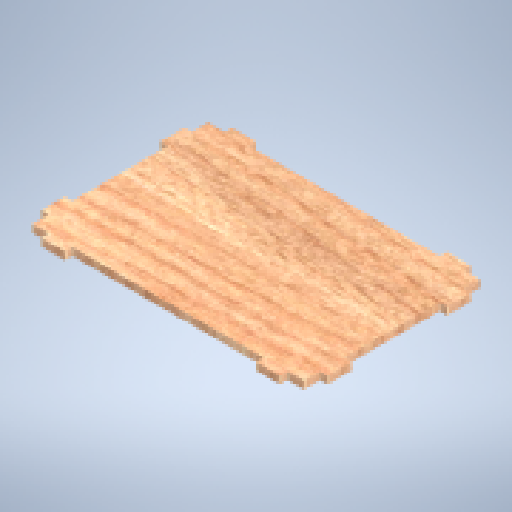
# Autodesk Inventor part: Bottom Panel
Saved by Autodesk Inventor 2023.1 (Build 271208000, 208)
## iProperties
Created: 2022-07-14
Part Number: Bottom Panel
Material: Wood (Birch)
Document SubType Name: Modeling
Designer: Eli
Density: 0.55 g/cm^3
Appearance: Birch - Natural Polished
Author: Eli
Autodesk Inventor part; units mm, degrees
ref_plane "YZ Plane" through (0, 0, 0) normal (1, 0, 0) x (0, 1, 0)
ref_plane "XZ Plane" through (0, 0, 0) normal (0, 1, 0) x (-1, 0, 0)
ref_plane "XY Plane" through (0, 0, 0) normal (0, 0, 1) x (1, 0, 0)
sketch "Sketch1" plane through (0, 0, 0) normal (0, 1, 0) x (-1, 0, 0)
  line L0 (0, 0) -> (152.4, 0)
  line L1 (152.4, 0) -> (152.4, 101.6)
  line L2 (152.4, 101.6) -> (0, 101.6)
  line L3 (0, 101.6) -> (0, 0)
  line L4 (152.4, 0) -> (139.7, 0)
  line L5 (139.7, 0) -> (139.7, 4)
  line L6 (139.7, 4) -> (152.4, 4)
  line L7 (152.4, 4) -> (152.4, 0)
  line L8 (0, 0) -> (12.7, 0)
  line L9 (12.7, 0) -> (12.7, 4)
  line L10 (12.7, 4) -> (0, 4)
  line L11 (0, 4) -> (0, 0)
  line L12 (127, 0) -> (25.4, 0)
  line L13 (25.4, 0) -> (25.4, 4)
  line L14 (25.4, 4) -> (127, 4)
  line L15 (127, 4) -> (127, 0)
  line L16 (152.4, 50.8) -> (0, 50.8)
  line L17 (139.7, 101.6) -> (139.7, 97.6)
  line L18 (139.7, 97.6) -> (152.4, 97.6)
  line L19 (12.7, 101.6) -> (12.7, 97.6)
  line L20 (12.7, 97.6) -> (0, 97.6)
  line L21 (25.4, 101.6) -> (25.4, 97.6)
  line L22 (25.4, 97.6) -> (127, 97.6)
  line L23 (127, 97.6) -> (127, 101.6)
  line L24 (152.4, 101.6) -> (148.4, 101.6)
  line L25 (148.4, 101.6) -> (148.4, 88.9)
  line L26 (148.4, 88.9) -> (152.4, 88.9)
  line L27 (152.4, 88.9) -> (152.4, 101.6)
  line L28 (152.4, 0) -> (148.4, 0)
  line L29 (148.4, 0) -> (148.4, 12.7)
  line L30 (148.4, 12.7) -> (152.4, 12.7)
  line L31 (152.4, 12.7) -> (152.4, 0)
  line L32 (152.4, 76.2) -> (148.4, 76.2)
  line L33 (148.4, 76.2) -> (148.4, 25.4)
  line L34 (148.4, 25.4) -> (152.4, 25.4)
  line L35 (152.4, 25.4) -> (152.4, 76.2)
  line L36 (76.2, 97.6) -> (76.2, 4)
  line L37 (4, 101.6) -> (4, 88.9)
  line L38 (4, 88.9) -> (0, 88.9)
  line L39 (4, 0) -> (4, 12.7)
  line L40 (4, 12.7) -> (0, 12.7)
  line L41 (0, 76.2) -> (4, 76.2)
  line L42 (4, 76.2) -> (4, 25.4)
  line L43 (4, 25.4) -> (0, 25.4)
  point P0 (12.7, 2)
  point P1 (25.4, 2)
  point P2 (150.4, 12.7)
  point P3 (150.4, 25.4)
  point P4 (150.4, 88.9)
  point P5 (150.4, 76.2)
  point P6 (148.4, 97.6)
  point P7 (4, 97.6)
  point P8 (4, 4)
  point P9 (25.4, 0)
  point P10 (148.4, 4)
  dimension "d0" = 152.4
  dimension "d1" = 101.6
  dimension "d2" = 12.7
  dimension "d3" = 4
  dimension "d4" = 12.7
  dimension "d5" = 4
  dimension "d6" = 4
  dimension "d7" = 12.7
  dimension "d8" = 12.7
  dimension "d9" = 4
  dimension "d10" = 12.7
  dimension "d11" = 4
  dimension "d12" = 12.7
  dimension "d13" = 4
  dimension "d14" = 12.7
  dimension "d15" = 12.7
  constraints: 88 end point, 20 symmetric about line, 14 parallel, 10 midpoint, 7 horizontal, 7 perpendicular, 2 point on line, 1 coincident
  measures "d0" distance of L2.end L1.end
  measures "d1" distance of L1.end L0.end
  measures "d2" distance of L5.end L6.end
  measures "d3" distance of L4.end L5.end
  measures "d4" distance of L10.end L9.end
  measures "d5" distance of L9.end L8.end
  measures "d6" distance of L12.end L13.end
  measures "d7" distance from line of L5.end L15
  measures "d8" distance of point (12.7, 2) point (25.4, 2)
  measures "d9" distance of L26.end L25.end
  measures "d10" distance of L25.end L24.end
  measures "d11" distance of L29.end L30.end
  measures "d12" distance of L28.end L29.end
  measures "d13" distance of L34.end L33.end
  measures "d14" distance of point (150.4, 12.7) point (150.4, 25.4)
  measures "d15" distance of point (150.4, 88.9) point (150.4, 76.2)
extrude "Extrusion1" add sketch "Sketch1" along normal blind 4 contours L9 L10 L39 L40 L3 L43 L42 L16 L36 L14 L13 L0 | L15 L14 L36 L16 L33 L34 L1 L30 L29 L6 L5 L0 | L3 L38 L37 L20 L19 L2 L21 L22 L36 L16 L42 L41 | L36 L22 L23 L2 L17 L18 L25 L26 L1 L32 L33 L16
ref_plane "Work Plane1" through (-127, 0, 50.8) normal (0, 0, 1) x (1, 0, 0)
body "Solid1"
